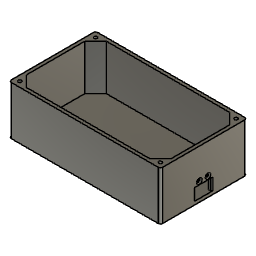
controllerBox v2 (Autodesk Fusion 360 design; units mm, degrees)
Autodesk Fusion 360 part; units mm, degrees
sketch "Sketch1" plane through (0, 0, 0) normal (0, 0, 1) x (1, 0, 0)
  line L0 (67, 37) -> (-67, 37)
  line L1 (-67, 37) -> (-67, -37)
  line L2 (-67, -37) -> (67, -37)
  line L3 (67, -37) -> (67, 37)
  line L4 (67, 37) -> (-67, -37) construction
  line L5 (-67, 37) -> (67, -37) construction
  line L6 (70, 40) -> (-70, 40)
  line L7 (-70, 40) -> (-70, -40)
  line L8 (-70, -40) -> (70, -40)
  line L9 (70, -40) -> (70, 40)
  line L10 (70, 40) -> (-70, -40) construction
  line L11 (-70, 40) -> (70, -40) construction
  dimension "d1" = 3
  dimension "d2" = 3
  dimension "d3" = 140
  dimension "d4" = 80
  constraint horizontal L0
  constraint perpendicular L0 L1
  constraint parallel L0 L2
  constraint parallel L1 L3
  constraint coincident L4 origin
  constraint coincident L5 origin
  constraint horizontal L6
  constraint perpendicular L6 L7
  constraint parallel L6 L8
  constraint parallel L7 L9
  constraint coincident L10 origin
  constraint coincident L11 origin
  measures "d1" distance of L3 L9
  measures "d2" distance of L0 L6
  measures "d3" distance of L6.start L6.end
  measures "d4" distance of L6.start L8.end
extrude "Extrude1" add sketch "Sketch1" along normal blind 45
sketch "Sketch2" plane through (0, 0, 0) normal (0, 0, 1) x (1, 0, 0)
  line L0 (-67, 37) -> (67, 37)
  line L1 (67, 37) -> (67, -37)
  line L2 (67, -37) -> (-67, -37)
  line L3 (-67, -37) -> (-67, 37)
  point P0 (-67, 37)
  point P1 (67, -37)
  constraint horizontal L0
  constraint vertical L1
  constraint horizontal L2
  constraint vertical L3
  constraint coincident P0 L0.start
  constraint coincident P1 L1.end
extrude "Extrude2" add sketch "Sketch2" along normal blind 3
sketch "Sketch3" plane through (0, 0, 3) normal (0, 0, 1) x (-1, 0, 0)
  line L0 (67, 37) -> (-67, 37)
  line L1 (-67, 37) -> (-67, -37)
  line L2 (-67, -37) -> (67, -37)
  line L3 (67, -37) -> (67, 37)
  line L4 (57, -37) -> (67, -27)
  line L5 (67, -27) -> (67, -37)
  line L6 (57, -37) -> (67, -37)
  dimension "d11" = 10
  dimension "d12" = 10
  constraint coincident L2 L4.start
  constraint coincident L3 L4.end
  constraint coincident L2.end L3.start
  measures "d11" distance of L4.start L2.end
  measures "d12" distance of L4.end L2.end
extrude "Extrude3" add sketch "Sketch3" along normal up to surface (42 mm away) contours L2 L3 L4 L5 L6
sketch "Sketch5" plane through (0, 0, 45) normal (0, 0, 1) x (-1, 0, 0)
  line L0 (-67, -37) -> (-67, 37)
  line L1 (-67, 37) -> (67, 37)
  line L2 (67, 37) -> (67, -27)
  line L3 (67, -27) -> (57, -37)
  line L4 (57, -37) -> (-67, -37)
  line L5 (-70, 40) -> (-70, -40)
  line L6 (-70, -40) -> (70, -40)
  line L7 (70, -40) -> (70, 40)
  line L8 (70, 40) -> (-70, 40)
  circle A0 centre (65, -35) radius 1.5
  line L9 (0, -1.75) -> (0, -22.5)
  line L10 (-1.75, 0) -> (-22.5, 0)
  dimension "d18" = 3
  dimension "d19" = 65
  dimension "d20" = 35
  measures "d18" diameter of A0
  measures "d19" distance of A0.centre L9
  measures "d20" distance of A0.centre L10
extrude "Extrude5" cut sketch "Sketch5" against normal blind 20 contours A0
mirror "Mirror1" about plane through (0, 0, 0) normal (1, 0, 0) of "Extrude3", "Extrude5"
mirror "Mirror2" about plane through (0, 0, 0) normal (0, 1, 0) of "Extrude3", "Extrude5", "Mirror1"
sketch "Sketch6" plane through (67, 0, 0) normal (-1, 0, 0) x (0, -1, 0)
  line L0 (27, 3) -> (27, 45)
  line L1 (27, 45) -> (-27, 45)
  line L2 (-27, 45) -> (-27, 3)
  line L3 (-27, 3) -> (27, 3)
  line L4 (7.5, 3) -> (-7.5, 3)
  line L5 (-7.5, 3) -> (-7.5, 13)
  line L6 (-7.5, 13) -> (7.5, 13)
  line L7 (7.5, 13) -> (7.5, 3)
  line L8 (7.5, 3) -> (-7.5, 13) construction
  line L9 (-7.5, 3) -> (7.5, 13) construction
  line L10 (-27, 15.2846) -> (0, 15.2846) construction
  line L11 (0, 15.2846) -> (27, 15.2846) construction
  circle A0 centre (-4, 17) radius 1.5
  line L12 (0, 2.5) -> (0, 20)
  circle A1 centre (4, 17) radius 1.5
  point P0 (0, 8)
  dimension "d27" = 10
  dimension "d28" = 15
  dimension "d29" = 3
  dimension "d30" = 4
  dimension "d31" = 4
  constraint horizontal L4
  constraint perpendicular L4 L5
  constraint parallel L4 L6
  constraint parallel L5 L7
  constraint coincident L3 L4.start
  constraint coincident L8 P0
  constraint coincident L9 P0
  constraint coincident L2 L10.start
  constraint perpendicular L2 L10
  constraint coincident L0 L11.end
  constraint perpendicular L0 L11
  constraint equal L10 L11
  constraint vertical P0 L10.end
  constraint symmetric A0 L12 A1
  measures "d27" distance of L4.start L6.end
  measures "d28" distance of L5.end L6.end
  measures "d29" diameter of A0
  measures "d30" horizontal distance of L10.end A0.centre
  measures "d31" distance of L6 A0.centre
extrude "Extrude6" cut sketch "Sketch6" along normal mid plane 20 contours L3 L4 L6 L7 L12 | L3 L4 L5 L6 L12 | A0 | A1
fillet "Fillet1" radius 2 4 edges at (70, -40, 22.5) (70, 40, 22.5) (-70, 40, 22.5) (-70, -40, 22.5)
fillet "Fillet2" radius 1 5 edges at (70, 0, 13) (70, -7.5, 8) (70, 7.5, 8) (70, 5.3985, 16.4576) (67, 5.3985, 17.5424) 1 faces at (68, -5.4925, 16.8506)
